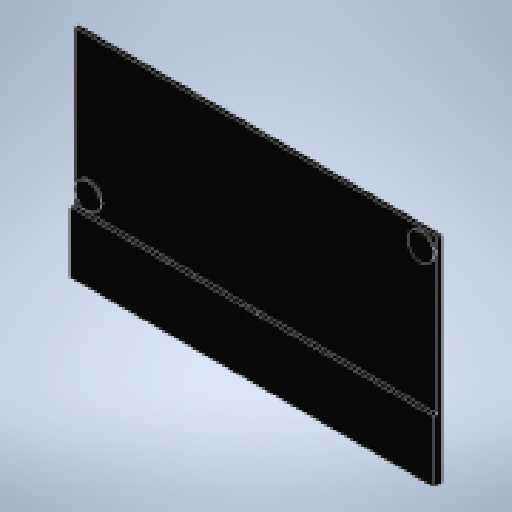
# Autodesk Inventor part: монитор
Saved by Autodesk Inventor 2023.1 (Build 271208000, 208)
## iProperties
Created: 2025-02-04
Part Number: монитор
Material: Типовые
Document SubType Name: Modeling
Designer: baranovaem
Density: 1 g/cm^3
Appearance: Черный
Author: baranovaem
Autodesk Inventor part; units mm, degrees
ref_plane "YZ Plane" through (0, 0, 0) normal (1, 0, 0) x (0, 1, 0)
ref_plane "XZ Plane" through (0, 0, 0) normal (0, 1, 0) x (-1, 0, 0)
ref_plane "XY Plane" through (0, 0, 0) normal (0, 0, 1) x (1, 0, 0)
sketch "Эскиз1" plane through (0, 0, 0) normal (0, 0, 1) x (1, 0, 0)
  line L0 (-177.5, 105) -> (177.5, 105)
  line L1 (177.5, 105) -> (177.5, -105)
  line L2 (177.5, -105) -> (-177.5, -105)
  line L3 (-177.5, -105) -> (-177.5, 105)
  line L4 (-177.5, 105) -> (177.5, -105) construction
  line L5 (177.5, 105) -> (-177.5, -105) construction
  point P0 (0, 0)
  dimension "d0" = 355
  dimension "d1" = 210
  constraints: 12 end point, 2 midpoint, 2 parallel, 1 horizontal, 1 perpendicular
  measures "d0" distance of L1.end L2.end
  measures "d1" distance of L0.end L1.end
extrude "Выдавливание1" add sketch "Эскиз1" along normal blind 4
sketch "Эскиз2" plane through (0, 0, 4) normal (0, 0, 1) x (1, 0, 0)
  line L0 (-177.5, -105) -> (177.5, -105) projected
  line L1 (177.5, -105) -> (177.5, 105) projected
  line L2 (-177.5, -105) -> (177.5, -105)
  line L3 (177.5, -105) -> (177.5, -45)
  line L4 (177.5, -45) -> (-177.5, -45)
  line L5 (-177.5, -45) -> (-177.5, -105)
  point P0 (0, 0)
  dimension "d4" = 60
  constraints: 8 end point, 2 parallel, 1 horizontal, 1 perpendicular, 1 point on line
  measures "d4" distance between parallel lines of L0 L4
extrude "Выдавливание2" add sketch "Эскиз2" along normal blind 4
sketch "Эскиз3" plane through (0, 0, 4) normal (0, 0, 1) x (1, 0, 0)
  circle A0 centre (-162.5, 90) radius 15
  circle A1 centre (162.5, -30) radius 15
  line L0 (177.5, 105) -> (-177.5, 105) construction
  line L1 (-177.5, 105) -> (-177.5, -45) construction
  line L2 (177.5, -45) -> (-177.5, -45) construction
  line L3 (177.5, -45) -> (177.5, 105) construction
  circle A2 centre (-162.5, 90) radius 12.75
  circle A3 centre (162.5, -30) radius 12.75
  point P0 (0, 0)
  dimension "d14" = 30
  dimension "d15" = 30
  dimension "d16" = 25.5
  dimension "d17" = 25.5
  constraints: 4 centre point, 4 tangent, 2 coincident
  measures "d14" diameter of A0
  measures "d15" diameter of A1
  measures "d16" diameter of A2
  measures "d17" diameter of A3
extrude "Выдавливание3" add sketch "Эскиз3" along normal blind 2 contours A2 | A3
